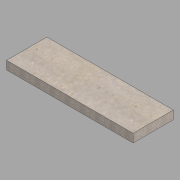
# Autodesk Inventor part: Retaining&exterior ST-3
Saved by Autodesk Inventor 2022.2 (Build 262287000, 287)
## iProperties
Created: 2021-10-22
Part Number: Retaining&exterior ST-3
Material: Limestone
Document SubType Name: Modeling
Designer: awelt
Density: 2.6 g/cm^3
Appearance: Kasota Gray
Mass: 193080 g
Surface Area: 18676.7 cm^2
Volume: 74261.7 cm^3
Author: awelt
Autodesk Inventor part; units mm, degrees
ref_plane "YZ Plane" through (0, 0, 0) normal (1, 0, 0) x (0, 1, 0)
ref_plane "XZ Plane" through (0, 0, 0) normal (0, 1, 0) x (-1, 0, 0)
ref_plane "XY Plane" through (0, 0, 0) normal (0, 0, 1) x (1, 0, 0)
sketch "Sketch1" plane through (0, 0, 0) normal (0, 1, 0) x (-1, 0, 0)
  line L0 (757.2756, -241.3) -> (-757.2756, -241.3)
  line L1 (-757.2756, -241.3) -> (-757.2756, 241.3)
  line L2 (-757.2756, 241.3) -> (757.2756, 241.3)
  line L3 (757.2756, 241.3) -> (757.2756, -241.3)
  line L4 (757.2756, -241.3) -> (-757.2756, 241.3) construction
  line L5 (-757.2756, -241.3) -> (757.2756, 241.3) construction
  point P0 (0, 0)
  dimension "d0" = 1514.5512
  dimension "d1" = 482.6
  constraints: 12 end point, 2 midpoint, 2 parallel, 1 horizontal, 1 perpendicular
  measures "d0" distance of L1.end L2.end
  measures "d1" distance of L0.end L1.end
extrude "Extrusion1" add sketch "Sketch1" along normal blind 101.6
body "Solid1"
